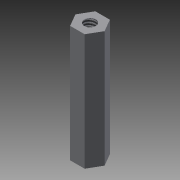
# Autodesk Inventor part: 000202
Saved by Autodesk Inventor 2015 (Build 190159000, 159)
## iProperties
Created: 2015-05-27
Part Number: 000202
Material: Generic
Document SubType Name: Modeling
Designer: Wesley
Density: 1 g/cm^3
Appearance: Default
Author: Wesley
Autodesk Inventor part; units mm, degrees
ref_plane "YZ Plane" through (0, 0, 0) normal (1, 0, 0) x (0, 1, 0)
ref_plane "XZ Plane" through (0, 0, 0) normal (0, 1, 0) x (-1, 0, 0)
ref_plane "XY Plane" through (0, 0, 0) normal (0, 0, 1) x (1, 0, 0)
sketch "Sketch2" plane through (0, 0, 0) normal (0, 1, 0) x (-1, 0, 0)
  line L0 (3.175, 0) -> (1.5875, -2.7496)
  line L1 (1.5875, -2.7496) -> (-1.5875, -2.7496)
  line L2 (-1.5875, -2.7496) -> (-3.175, 0)
  line L3 (-3.175, 0) -> (-1.5875, 2.7496)
  line L4 (-1.5875, 2.7496) -> (1.5875, 2.7496)
  line L5 (1.5875, 2.7496) -> (3.175, 0)
  point P0 (0, 0)
  point P1 (0, 0)
  dimension "d0" = 6.35
  dimension "d1" = 2.7496
  constraints: 12 end point, 1 coincident, 13 other
  measures "d0" distance of L2.end L0.start
  measures "d1" vertical distance of L1.end L2.end
extrude "Extrusion1" add sketch "Sketch2" along normal blind 25.4
sketch "Sketch3" plane through (0, 25.4, 0) normal (0, 1, 0) x (1, 0, 0)
  line L0 (-1.5875, 2.7496) -> (-3.175, 0) projected
  line L1 (-3.175, 0) -> (-1.5875, -2.7496) projected
  line L2 (-1.5875, -2.7496) -> (1.5875, -2.7496) projected
  line L3 (1.5875, -2.7496) -> (3.175, 0) projected
  line L4 (3.175, 0) -> (1.5875, 2.7496) projected
  line L5 (1.5875, 2.7496) -> (-1.5875, 2.7496) projected
  point P0 (0, 0)
hole "Hole1" at (0, 25.4, 0) direction (0, -1, 0) diameter 2.4892 end through all
body "Solid1"
